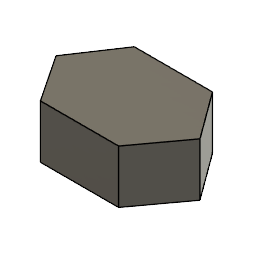
replay (Autodesk Fusion 360 design; units mm, degrees)
Autodesk Fusion 360 part; units mm, degrees
ref_plane "工作平面1" through (0, 20, 0) normal (0, 1, 0) x (0, 0, 1)
sketch "草图1" plane through (0, 20, 0) normal (0, 1, 0) x (1, 0, 0)
  line L0 (-5, -20) -> (5, -5)
  line L1 (5, -5) -> (30, -5)
  line L2 (30, -5) -> (41, -20)
  line L3 (41, -20) -> (30, -35)
  line L4 (30, -35) -> (5, -35)
  line L5 (5, -35) -> (-5, -20)
extrude "拉伸1" add sketch "草图1" against normal blind 17
